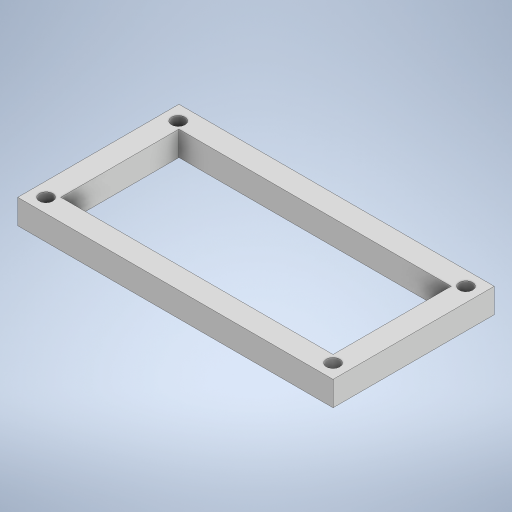
# Autodesk Inventor part: Buck 2
Saved by Autodesk Inventor 2024 (Build 280153000, 153)
## iProperties
Created: 2023-06-26
Part Number: Buck 2
Material: Genérico
Document SubType Name: Modeling
Designer: sergi
Density: 1 g/cm^3
Appearance: Valor por defecto
Author: sergi
Autodesk Inventor part; units mm, degrees
ref_plane "YZ Plane" through (0, 0, 0) normal (1, 0, 0) x (0, 1, 0)
ref_plane "XZ Plane" through (0, 0, 0) normal (0, 1, 0) x (-1, 0, 0)
ref_plane "XY Plane" through (0, 0, 0) normal (0, 0, 1) x (1, 0, 0)
sketch "Boceto1" plane through (0, 0, 0) normal (0, 1, 0) x (-1, 0, 0)
  line L0 (-25.625, -13.1) -> (25.625, -13.1)
  line L1 (25.625, -13.1) -> (25.625, 13.1)
  line L2 (25.625, 13.1) -> (-25.625, 13.1)
  line L3 (-25.625, 13.1) -> (-25.625, -13.1)
  line L4 (-25.625, -13.1) -> (25.625, 13.1) construction
  line L5 (25.625, -13.1) -> (-25.625, 13.1) construction
  line L6 (24.425, -11.9) -> (-24.425, -11.9)
  line L7 (-24.425, -10.8) -> (-24.425, 10.8)
  circle A0 centre (23.325, 10.8) radius 1.1
  circle A1 centre (-23.325, 10.8) radius 1.1
  circle A2 centre (-23.325, -10.8) radius 1.1
  circle A3 centre (23.325, -10.6888) radius 1.1
  line L8 (-24.425, 11.9) -> (-23.2777, 11.9)
  line L9 (23.2777, 11.9) -> (23.325, 11.9)
  line L10 (-22.125, 9.6) -> (22.125, 9.6)
  line L11 (22.125, 9.6) -> (22.125, -9.6)
  line L12 (22.125, -9.6) -> (-22.125, -9.6)
  line L13 (-22.125, -9.6) -> (-22.125, 9.6)
  point P0 (0, 0)
  dimension "d3" = 2.2
  dimension "d4" = 2.2
  dimension "d5" = 2.2
  dimension "d0" = 51.25
  dimension "d1" = 26.2
  dimension "d6" = 2.2
  dimension "d7" = 3.5
  constraints: 28 end point, 6 horizontal, 6 parallel, 2 horizontal alignment, 2 midpoint, 2 perpendicular, 2 point on line, 2 vertical, 1 centre point, 1 tangent, 1 vertical alignment, 9 other
  measures "d0" distance of L2.end L1.end
  measures "d1" distance of L1.end L0.end
  measures "d6" diameter of A3
  measures "d7" distance between parallel lines of L2 L10
extrude "Extrusión1" add sketch "Boceto1" along normal blind 4
